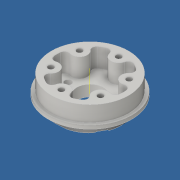
# Autodesk Inventor part: GripperRot
Saved by Autodesk Inventor 2016 (Build 200138000, 138)
## iProperties
Created: 2016-03-29
Part Number: GripperRot
Material: ABS-Kunststoff
Document SubType Name: Modeling
Designer: 4ndreas
Density: 1.06 g/cm^3
Appearance: Glatt - weiß
Mass: 7.40024 g
Surface Area: 53.7002 cm^2
Volume: 6.98136 cm^3
Author: 4ndreas
Autodesk Inventor part; units mm, degrees
ref_plane "YZ Plane" through (0, 0, 0) normal (1, 0, 0) x (0, 1, 0)
ref_plane "XZ Plane" through (0, 0, 0) normal (0, 1, 0) x (-1, 0, 0)
sketch "Skizze1" plane through (0, 0, 0) normal (0, 0, 1) x (1, 0, 0)
  circle A0 centre (0, 0) radius 19
  circle A1 centre (0, 0) radius 15
  dimension "d0" = 38
  dimension "d1" = 30
  constraints: 2 centre point, 2 coincident
  measures "d0" diameter of A0
  measures "d1" diameter of A1
extrude "Extrusion1" add sketch "Skizze1" along normal blind 1.6
sketch "Skizze2" plane through (0, 0, 1.6) normal (0, 0, 1) x (1, 0, 0)
  circle A0 centre (0, 0) radius 15
  circle A1 centre (0, 0) radius 19
  circle A2 centre (0, 0) radius 17.5
  dimension "d4" = 35
  constraints: 3 centre point, 1 coincident
  measures "d4" diameter of A2
extrude "Extrusion2" add sketch "Skizze2" along normal blind 7 contours A2
sketch "Skizze3" plane through (0, 0, 0) normal (0, 0, -1) x (-1, 0, 0)
  circle A0 centre (0, 0) radius 15
  circle A1 centre (0, 0) radius 17.5
  constraints: 2 centre point
extrude "Extrusion3" add sketch "Skizze3" along normal blind 5 contours A0 | A1
sketch "Skizze4" plane through (0, 0, -5) normal (0, 0, -1) x (-1, 0, 0)
  circle A0 centre (0, 0) radius 6
  dimension "d9" = 12
  constraints: 1 centre point, 1 coincident
  measures "d9" diameter of A0
extrude "Extrusion4" cut sketch "Skizze4" against normal through all
chamfer "Fase1" [suppressed]
chamfer "Fase2" [suppressed]
sketch "Skizze5" plane through (0, 0, -5) normal (0, 0, -1) x (-1, 0, 0)
  line L0 (0, 0) -> (0, 14.7265)
  constraints: 2 end point, 1 vertical
ref_plane "Arbeitsebene1" through (0, 0, -5) normal (-1, 0, 0) x (0, 1, 0)
sketch "Skizze6" plane through (0, 0, -5) normal (-1, 0, 0) x (0, 1, 0)
  line L0 (-19, -6.6) -> (-19, -5) projected
  line L1 (-19, -5) -> (-17.5, -5) projected
  line L2 (-17.5, -5) -> (-17.5, 0) projected
  line L3 (-17.5, 0) -> (-6, 0) projected
  line L4 (-6, 0) -> (-6, -5) projected
  line L5 (-6, -5) -> (-15, -5) projected
  line L6 (-15, -5) -> (-15, -13.6) projected
  line L7 (-15, -13.6) -> (-17.5, -13.6) projected
  line L8 (-17.5, -13.6) -> (-17.5, -6.6) projected
  line L9 (-17.5, -6.6) -> (-19, -6.6) projected
  line L10 (19, -5) -> (19, -6.6) projected
  line L11 (19, -6.6) -> (17.5, -6.6) projected
  line L12 (17.5, -6.6) -> (17.5, -13.6) projected
  line L13 (17.5, -13.6) -> (15, -13.6) projected
  line L14 (15, -13.6) -> (15, -5) projected
  line L15 (15, -5) -> (6, -5) projected
  line L16 (6, -5) -> (6, 0) projected
  line L17 (6, 0) -> (17.5, 0) projected
  line L18 (17.5, 0) -> (17.5, -5) projected
  line L19 (17.5, -5) -> (19, -5) projected
  line L20 (19, -5) -> (14, 0)
  line L21 (19, -5) -> (15, -5)
  line L22 (17.5, -5) -> (17.5, -3.5)
  line L23 (14, 0) -> (17.5, 0)
  line L24 (17.5, -3.5) -> (17.5, 0)
  line L25 (0, 2.8) -> (0, -16.8) projected
  point P0 (0, -5)
  dimension "d19" = 45
  constraints: 10 end point, 3 point on line, 2 collinear, 1 horizontal
  measures "d19" angle of L19 L20
revolve "Umdrehung1" add sketch "Skizze6" angle 360 about axis through (0, 0, -5) along (0, 0, 1) contours L19 L18 L20
revolve "Umdrehung2" cut sketch "Skizze6" angle 360 about axis through (0, 0, -5) along (0, 0, 1) contours L20 L17 L18
sketch "Skizze7" plane through (0, 0, 0) normal (0, 0, 1) x (1, 0, 0)
  circle A0 centre (0, 0) radius 10 construction
  line L0 (10, 0) -> (-10, 0) construction
  dimension "d22" = 20
  constraints: 2 coincident, 2 end point, 2 point on circle, 1 centre point, 1 horizontal, 1 midpoint
  measures "d22" diameter of A0
hole "Bohrung1" at (10, 0, 0) at (-10, 0, 0) direction (0, 0, -1) diameter 3 end through all
sketch "Skizze8" plane through (0, 0, 8.6) normal (0, 0, 1) x (1, 0, 0)
  circle A0 centre (0, 0) radius 13 construction
  line L0 (11.2583, 6.5) -> (11.2583, -6.5) construction
  line L1 (11.2583, -6.5) -> (0, -13) construction
  line L2 (0, -13) -> (-11.2583, -6.5) construction
  line L3 (-11.2583, -6.5) -> (-11.2583, 6.5) construction
  line L4 (-11.2583, 6.5) -> (0, 13) construction
  line L5 (0, 13) -> (11.2583, 6.5) construction
  circle A1 centre (11.2583, 6.5) radius 3.5
  circle A2 centre (0, 0) radius 15 construction
  circle A3 centre (0, 0) radius 17.5 construction
  circle A4 centre (0, 13) radius 3.5
  circle A5 centre (-11.2583, 6.5) radius 3.5
  circle A6 centre (-11.2583, -6.5) radius 3.5
  circle A7 centre (0, -13) radius 3.5
  circle A8 centre (11.2583, -6.5) radius 3.5
  dimension "d30" = 26
  dimension "d31" = 7
  constraints: 12 coincident, 12 end point, 7 centre point, 5 equal radius, 2 point on circle, 1 vertical, 13 other
  measures "d30" diameter of A0
  measures "d31" diameter of A1
extrude "Extrusion5" add sketch "Skizze8" against normal up to surface (8.6 mm away)
hole "Bohrung2" at (11.2583, 6.5, 8.6) at (11.2583, -6.5, 8.6) at (0, -13, 8.6) at (-11.2583, 6.5, 8.6) at (0, 13, 8.6) at (-11.2583, -6.5, 8.6) direction (0, 0, -1) diameter 2.5 end through all
fillet "Rundung1" radius 2 12 edges at (-14.2501, 4.6835, 4.3) (-11.1811, 9.9991, 4.3) (-11.1811, -9.9991, 4.3) (-14.2501, -4.6835, 4.3) (3.069, -14.6827, 4.3) (-3.069, -14.6827, 4.3) (11.1811, -9.9991, 4.3) (14.2501, -4.6835, 4.3) (14.2501, 4.6835, 4.3) (11.1811, 9.9991, 4.3) (-3.069, 14.6827, 4.3) (3.069, 14.6827, 4.3)
sketch "Skizze9" plane through (0, 0, -5) normal (0, 0, -1) x (-1, 0, 0)
  circle A0 centre (0, 0) radius 6 projected
  arc A1 (-0.778, 13.9784) -> (0.778, 13.9784) centre (0, 13) ccw projected
  arc A2 (-0.778, 13.9784) -> (-11.7166, 7.663) centre (0, 0) ccw projected
  arc A3 (-12.4946, 6.3154) -> (-11.7166, 7.663) centre (-11.2583, 6.5) ccw projected
  arc A4 (-12.4946, 6.3154) -> (-12.4946, -6.3154) centre (0, 0) ccw projected
  arc A5 (-11.7166, -7.663) -> (-12.4946, -6.3154) centre (-11.2583, -6.5) ccw projected
  arc A6 (-11.7166, -7.663) -> (-0.778, -13.9784) centre (0, 0) ccw projected
  arc A7 (0.778, -13.9784) -> (-0.778, -13.9784) centre (0, -13) ccw projected
  arc A8 (0.778, -13.9784) -> (11.7166, -7.663) centre (0, 0) ccw projected
  arc A9 (12.4946, -6.3154) -> (11.7166, -7.663) centre (11.2583, -6.5) ccw projected
  arc A10 (12.4946, -6.3154) -> (12.4946, 6.3154) centre (0, 0) ccw projected
  arc A11 (11.7166, 7.663) -> (12.4946, 6.3154) centre (11.2583, 6.5) ccw projected
  arc A12 (11.7166, 7.663) -> (0.778, 13.9784) centre (0, 0) ccw projected
  circle A13 centre (10, 0) radius 1.5 projected
  circle A14 centre (-10, 0) radius 1.5 projected
  line L0 (-12.846, -3.75) -> (-9.6706, -3.75)
  line L1 (-9.6706, -3.75) -> (-8.0829, -6.5)
  line L2 (-8.0829, -6.5) -> (-9.6706, -9.25)
  line L3 (-9.6706, -9.25) -> (-12.846, -9.25)
  line L4 (-12.846, -9.25) -> (-14.4338, -6.5)
  line L5 (-14.4338, -6.5) -> (-12.846, -3.75)
  line L6 (3.1754, 13) -> (1.5877, 10.25)
  line L7 (1.5877, 10.25) -> (-1.5877, 10.25)
  line L8 (-1.5877, 10.25) -> (-3.1754, 13)
  line L9 (-3.1754, 13) -> (-1.5877, 15.75)
  line L10 (-1.5877, 15.75) -> (1.5877, 15.75)
  line L11 (1.5877, 15.75) -> (3.1754, 13)
  line L12 (9.6706, 9.25) -> (12.846, 9.25)
  line L13 (12.846, 9.25) -> (14.4338, 6.5)
  line L14 (14.4338, 6.5) -> (12.846, 3.75)
  line L15 (12.846, 3.75) -> (9.6706, 3.75)
  line L16 (9.6706, 3.75) -> (8.0829, 6.5)
  line L17 (8.0829, 6.5) -> (9.6706, 9.25)
  line L18 (8.0829, -6.5) -> (9.6706, -3.75)
  line L19 (9.6706, -3.75) -> (12.846, -3.75)
  line L20 (12.846, -3.75) -> (14.4338, -6.5)
  line L21 (14.4338, -6.5) -> (12.846, -9.25)
  line L22 (12.846, -9.25) -> (9.6706, -9.25)
  line L23 (9.6706, -9.25) -> (8.0829, -6.5)
  line L24 (1.5877, -10.25) -> (3.1754, -13)
  line L25 (3.1754, -13) -> (1.5877, -15.75)
  line L26 (1.5877, -15.75) -> (-1.5877, -15.75)
  line L27 (-1.5877, -15.75) -> (-3.1754, -13)
  line L28 (-3.1754, -13) -> (-1.5877, -10.25)
  line L29 (-1.5877, -10.25) -> (1.5877, -10.25)
  line L30 (0, -13) -> (0, 13) construction
  line L31 (-11.2583, -6.5) -> (11.2583, 6.5) construction
  line L32 (11.2583, -6.5) -> (-11.2583, 6.5) construction
  line L33 (-12.846, 9.25) -> (-9.6706, 9.25)
  line L34 (-9.6706, 9.25) -> (-8.0829, 6.5)
  line L35 (-8.0829, 6.5) -> (-9.6706, 3.75)
  line L36 (-9.6706, 3.75) -> (-12.846, 3.75)
  line L37 (-12.846, 3.75) -> (-14.4338, 6.5)
  line L38 (-14.4338, 6.5) -> (-12.846, 9.25)
  dimension "d42" = 5.5
  constraints: 78 end point, 7 coincident, 5 equal length, 5 perpendicular, 1 point on line, 1 vertical, 78 other
  measures "d42" distance between parallel lines of L25 L28
extrude "Extrusion6" cut sketch "Skizze9" against normal blind 5 contours A2 L9 L10 L11 A12 A1 | A1 A12 L11 L6 L7 L8 L9 A2 | L33 L34 L35 L36 L37 A4 A3 A2 | A2 A3 A4 L37 L38 L33 | L12 L13 L14 A10 A11 A12 | A12 A11 A10 L14 L15 L16 L17 L12 | L5 L0 L1 L2 L3 A6 A5 A4 | A4 A5 A6 L3 L4 L5 | L20 L21 L22 A8 A9 A10 | A10 A9 A8 L22 L23 L18 L19 L20 | L27 L28 L29 L24 L25 A8 A7 A6 | A6 A7 A8 L25 L26 L27
sketch "Skizze10" plane through (0, 0, 0) normal (0, 0, -1) x (-1, 0, 0)
  circle A0 centre (11.2583, -6.5) radius 1.25 projected
  circle A1 centre (0, -13) radius 1.25 projected
  circle A2 centre (0, -13) radius 1.25 projected
  circle A3 centre (-11.2583, -6.5) radius 1.25 projected
  circle A4 centre (-11.2583, -6.5) radius 1.25 projected
  circle A5 centre (-11.2583, 6.5) radius 1.25 projected
  circle A6 centre (0, 13) radius 1.25 projected
  circle A7 centre (0, 13) radius 1.25 projected
  circle A8 centre (11.2583, 6.5) radius 1.25 projected
  circle A9 centre (11.2583, 6.5) radius 1.25 projected
  point P0 (0, 0)
extrude "Extrusion7" add sketch "Skizze10" against normal blind 0.2
